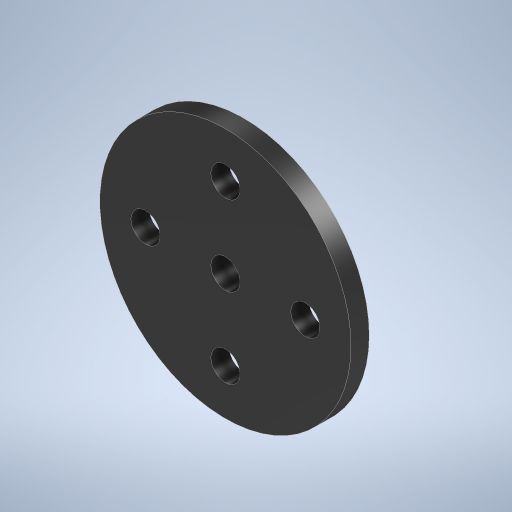
# Autodesk Inventor part: servo horn wide
Saved by Autodesk Inventor 2023 (Build 270158000, 158)
## iProperties
Created: 2023-03-24
Part Number: servo horn wide
Material: 一般
Document SubType Name: Modeling
Designer: zegi
Density: 1 g/cm^3
Appearance: 光沢 - 黒
Author: zegi
Autodesk Inventor part; units mm, degrees
ref_plane "YZ Plane" through (0, 0, 0) normal (1, 0, 0) x (0, 1, 0)
ref_plane "XZ Plane" through (0, 0, 0) normal (0, 1, 0) x (-1, 0, 0)
ref_plane "XY Plane" through (0, 0, 0) normal (0, 0, 1) x (1, 0, 0)
sketch "スケッチ1" plane through (0, 0, 0) normal (0, 0, 1) x (1, 0, 0)
  circle A0 centre (0, 0) radius 13.75
  line L0 (0, 13.75) -> (0, -13.75) construction
  line L1 (13.75, 0) -> (-13.75, 0) construction
  circle A1 centre (0, 0) radius 5
  point P0 (0, 8.75)
  point P1 (0, -8.75)
  point P2 (8.75, 0)
  point P3 (-8.75, 0)
  dimension "d0" = 27.5
  dimension "d1" = 17.5
  dimension "d2" = 17.5
  dimension "d3" = 10
  constraints: 4 end point, 4 midpoint, 4 point on circle, 4 point on line, 3 coincident, 2 centre point, 2 symmetric about line, 1 perpendicular, 1 vertical
  measures "d0" diameter of A0
  measures "d1" distance of point (0, -8.75) point (0, 8.75)
  measures "d2" distance of point (-8.75, 0) point (8.75, 0)
  measures "d3" diameter of A1
extrude "押し出し1" add sketch "スケッチ1" along normal blind 2 contours A0 | A1
extrude "押し出し2" add sketch "スケッチ1" against normal blind 4.7 contours A1
hole "穴1" at (0, 0, 0) at (0, 8.75, 0) at (0, -8.75, 0) at (8.75, 0, 0) at (-8.75, 0, 0) direction (0, 0, -1) diameter 3.2 depth 8 tip angle 118
hole "穴2" at (-8.75, 0, 0) at (0, 8.75, 0) at (8.75, 0, 0) at (0, -8.75, 0) at (0, 0, 0) direction (0, 0, 1) diameter 3.2 depth 8 tip angle 118
sketch "スケッチ3" plane through (0, 0, 2) normal (0, 0, 1) x (1, 0, 0)
  circle A0 centre (0, -8.75) radius 1.6 projected
  circle A1 centre (0, 8.75) radius 1.6 projected
  circle A2 centre (-8.75, 0) radius 1.6 projected
  circle A3 centre (8.75, 0) radius 1.6 projected
  circle A4 centre (0, 0) radius 1.6 projected
  circle A5 centre (0, 0) radius 13.75 projected
equation "\"d2\" = d1"
